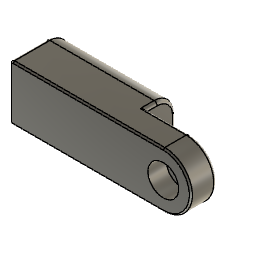
motor-holder (Autodesk Fusion 360 design; units mm, degrees)
Autodesk Fusion 360 part; units mm, degrees
sketch "Sketch1" plane through (-6.6733, 19.3, -27.7832) normal (0, 1, 0) x (-1, 0, 0)
  circle A0 centre (-1.5233, 27.7832) radius 2.25
  circle A1 centre (-1.5233, 27.7832) radius 0.8
  circle A2 centre (-1.5233, 27.7832) radius 2.5
  circle A3 centre (-1.5233, 27.7832) radius 0.8
  circle A4 centre (-1.5233, 27.7832) radius 4.5
  line L0 (-1.5233, 27.7832) -> (16.4767, 27.7832) construction
  line L1 (23.4767, 32.2832) -> (-1.5233, 32.2832)
  line L2 (23.4767, 23.2832) -> (-1.5233, 23.2832)
  line L3 (23.4767, 32.2832) -> (23.4767, 23.2832)
  line L4 (5.4767, 32.2832) -> (5.4767, 23.2832)
  dimension "d1" = 18
  dimension "d4" = 9
  dimension "d7" = 9
  dimension "d8" = 25
  dimension "d9" = 18
  constraint concentric A2 A4
  constraint coincident A0.centre A1.centre
  constraint horizontal L0
  constraint coincident A4 L1.end
  constraint coincident A4 L2.end
  constraint tangent A4 L1
  constraint tangent A4 L2
  constraint perpendicular L2 L3
  constraint coincident L1 L4.start
  constraint coincident L2 L4.end
  constraint perpendicular L2 L4
  measures "d1" distance of A0.centre L0.end
  measures "d4" diameter of A4
  measures "d7" distance of L1.start L2.start
  measures "d8" distance of L1.start L1.end
  measures "d9" distance of L3 L4
extrude "Extrude1" add sketch "Sketch1" against normal blind 3 contours A4 | A4 L1 L2 L4 | L1 L2 L3 L4
extrude "Extrude2" add sketch "Sketch1" along normal blind 6 contours L1 L2 L3 L4
sketch "Sketch2" plane through (-30.15, 0, 0) normal (-1, 0, 0) x (0, -1, 0)
  line L0 (-25.3, -4.5) -> (-16.3, -4.5)
  line L1 (-16.3, -4.5) -> (-16.3, 4.5)
  line L2 (-16.3, 4.5) -> (-25.3, 4.5)
  line L3 (-25.3, 4.5) -> (-25.3, -4.5)
  line L4 (-16.3, 0) -> (-25.3, 0) construction
  line L5 (-20.8, 4.5) -> (-20.8, -4.5) construction
  circle A0 centre (-20.8, 0) radius 3.1
  dimension "d12" = 6.2
  constraint midpoint L1 L4.start
  constraint midpoint L3 L4.end
  constraint midpoint L2 L5.start
  constraint midpoint L0 L5.end
  constraint midpoint L5 A0.centre
  measures "d12" diameter of A0
extrude "Extrude3" cut sketch "Sketch2" against normal blind 15 contours A0
fillet "Fillet1" radius 3 2 edges at (-21.15, 25.3, 4.5) (-21.15, 25.3, -4.5)
fillet "Fillet7" radius 0.5 5 edges at (-30.15, 19.3, -4.5) (-30.15, 24.4213, -3.6213) (-30.15, 25.3, 0) (-30.15, 24.4213, 3.6213) (-30.15, 19.3, 4.5)
chamfer "Chamfer1" distance 0.25 angle 45 6 edges at (-17.4, 16.3, -4.5) (-0.65, 16.3, 0) (-17.4, 16.3, 4.5) (-30.0036, 16.3, 4.3536) (-30.15, 16.3, 0) (-30.0036, 16.3, -4.3536)
sketch "Sketch3" plane through (-12.15, 0, 0) normal (1, 0, 0) x (0, 1, 0)
  line L0 (19.3, 4.5) -> (19.3, -4.5)
  circle A0 centre (22.8, 0) radius 1
  arc A1 (22.3, -4.5) -> (25.3, -1.5) centre (22.3, -1.5) ccw
  line L1 (25.3, -1.5) -> (25.3, 1.5)
  arc A2 (25.3, 1.5) -> (22.3, 4.5) centre (22.3, 1.5) ccw
  line L2 (22.3, 4.5) -> (19.3, 4.5)
  line L3 (19.3, -4.5) -> (22.3, -4.5)
  line L4 (22.3, 4.5) -> (22.3, -4.5) construction
  line L5 (22.8, 4.458) -> (22.8, -4.458) construction
  line L6 (25.3, 0) -> (19.3, 0) construction
  dimension "d22" = 2
  dimension "d30" = 0.5
  constraint coincident A2.end L2.start
  constraint coincident A1.start L3.end
  constraint coincident A2 L5.start
  constraint coincident A1 L5.end
  constraint vertical L5
  constraint midpoint L1 L6.start
  constraint midpoint L0 L6.end
  constraint coincident A0.centre L5
  constraint coincident A0.centre L6
  measures "d22" diameter of A0
  measures "d30" distance of L4 L5
extrude "Extrude4" cut sketch "Sketch3" against normal up to surface (3 mm away) contours A0
sketch "Sketch4" plane through (0, 19.3, 0) normal (0, 1, 0) x (-1, 0, 0)
  circle A0 centre (5.15, 0) radius 2.5
  circle A1 centre (5.15, 0) radius 0.85
  line L0 (12.15, 4.5) -> (5.15, 4.5)
  arc A2 (5.15, 4.5) -> (5.15, -4.5) centre (5.15, 0) ccw
  line L1 (5.15, -4.5) -> (12.15, -4.5)
  line L2 (12.15, 4.5) -> (5.15, 4.5)
  arc A3 (5.15, 4.5) -> (5.15, -4.5) centre (5.15, 0) ccw
  line L3 (5.15, -4.5) -> (12.15, -4.5)
  circle A4 centre (5.15, 0) radius 2.5
  line L4 (12.15, 1.5) -> (12.15, -1.5)
  line L5 (12.15, 1.5) -> (12.15, 4.5)
  line L6 (12.15, -4.5) -> (12.15, -1.5)
  dimension "d25" = 1.7
  measures "d25" diameter of A1
extrude "Extrude6" add sketch "Sketch4" along normal blind 1.25 contours A0 A4 | L0 A2 L1 L2 A3 L3 L4 L5 L6
fillet "Fillet8" radius 0.5 8 edges at (-8.65, 20.55, 4.5) (-0.65, 20.55, 0) (-8.65, 20.55, -4.5) (-12.15, 21.425, 4.5) (-12.15, 24.4213, 3.6213) (-12.15, 25.3, 0) (-12.15, 24.4213, -3.6213) (-12.15, 21.425, -4.5)
equation "d4 = 6 mm + wall_thickness"
equation "d9 = 15 mm + 3 mm"
equation "wall_thickness = 3 mm"
